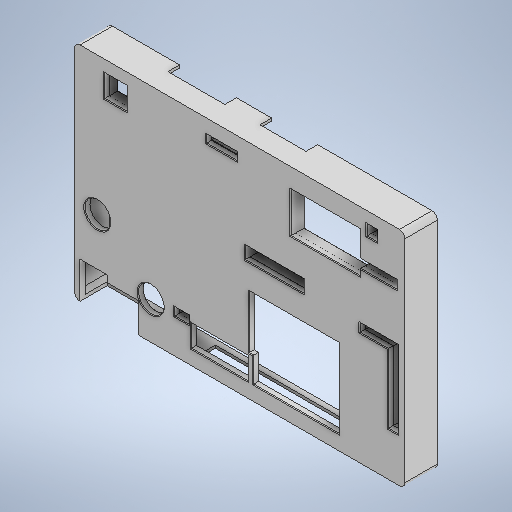
# Autodesk Inventor part: tampa_KiiRA
Saved by Autodesk Inventor 2026.3 (Build 303398000, 398)
## iProperties
Created: 2026-05-20
Part Number: tampa_KiiRA
Material: Genérico
Document SubType Name: Modeling
Designer: franciscowilke
Density: 1 g/cm^3
Appearance: Padrão
Author: franciscowilke
Autodesk Inventor part; units mm, degrees
ref_plane "YZ Plane" through (0, 0, 0) normal (1, 0, 0) x (0, 1, 0)
ref_plane "XZ Plane" through (0, 0, 0) normal (0, 1, 0) x (-1, 0, 0)
ref_plane "XY Plane" through (0, 0, 0) normal (0, 0, 1) x (1, 0, 0)
sketch "Esboço2" plane through (0, 0, 0) normal (0, 0, 1) x (1, 0, 0)
  line L0 (60.2596, 45.3747) -> (-61.7404, 45.3747)
  line L1 (-61.7404, 45.3747) -> (-61.7404, -36.6253)
  line L2 (-61.7404, -36.6253) -> (60.2596, -36.6253)
  line L3 (60.2596, -36.6253) -> (60.2596, 45.3747)
  line L4 (60.2596, 45.3747) -> (-61.7404, -36.6253) construction
  line L5 (-61.7404, 45.3747) -> (60.2596, -36.6253) construction
  point P0 (0, 0)
  dimension "d9" = 122
  dimension "d10" = 82
  constraints: 12 end point, 2 parallel, 1 horizontal, 1 perpendicular
  measures "d9" distance of L2.end L1.end
  measures "d10" distance of L1.end L0.end
extrude "Extrusão6" add sketch "Esboço2" against normal blind 12
sketch "Esboço11" plane through (0, 0, -12) normal (0, 0, -1) x (-1, 0, 0)
  line L0 (61.7404, -36.6253) -> (61.7404, 45.3747) construction
  line L1 (61.7404, 45.3747) -> (-60.2596, 45.3747) construction
  line L2 (-60.2596, 45.3747) -> (-60.2596, -36.6253) construction
  line L3 (-60.2596, -36.6253) -> (61.7404, -36.6253) construction
  line L4 (-60.2596, 45.3747) -> (61.7404, 45.3747)
  line L5 (61.7404, 45.3747) -> (61.7404, -36.6253)
  line L6 (61.7404, -36.6253) -> (-60.2596, -36.6253)
  line L7 (-60.2596, -36.6253) -> (-60.2596, 45.3747)
  line L8 (-59.2596, 44.3747) -> (60.7404, 44.3747)
  line L9 (60.7404, 44.3747) -> (60.7404, -35.6253)
  line L10 (60.7404, -35.6253) -> (-59.2596, -35.6253)
  line L11 (-59.2596, -35.6253) -> (-59.2596, 44.3747)
  point P0 (0, 0)
  dimension "d193" = 1
  constraints: 16 end point, 2 parallel, 1 horizontal, 1 perpendicular, 3 other
  measures "d193" distance between parallel lines of L1 L8
extrude "Extrusão8" cut sketch "Esboço11" against normal blind 10 contours L8 L9 L10 L11
fillet "Arredondamento3" radius 2 8 edges at (-60.7404, 44.3747, -7) (60.2596, -36.6253, -6) (-61.7404, -36.6253, -6) (-60.7404, -35.6253, -7) (-61.7404, 45.3747, -6) (60.2596, 45.3747, -6) (59.2596, 44.3747, -7) (59.2596, -35.6253, -7)
sketch "Esboço4" plane through (0, 0, 0) normal (0, 0, 1) x (1, 0, 0)
  line L0 (2.6091, -2.1634) -> (35.9721, -2.118)
  line L1 (53.9733, -20.4796) -> (53.9372, 5.0204)
  line L2 (53.9372, 5.0204) -> (43.5268, 5.0002)
  line L3 (22.8706, 7.0991) -> (1.1206, 7.0659)
  line L4 (1.1206, 7.0659) -> (1.1206, 11.8159)
  line L5 (1.1206, 11.8159) -> (22.8706, 11.8159)
  line L6 (22.8706, 11.8159) -> (22.8706, 7.0991)
  line L7 (17.9879, 23.1518) -> (43.7379, 23.1518)
  line L8 (43.7379, 23.1518) -> (43.7379, 25.5518)
  circle A0 centre (-53.3326, -5.722) radius 4.75
  arc A1 (-28.9083, -23.3517) -> (-38.3779, -23.3517) centre (-33.6431, -22.972) ccw
  line L9 (17.9879, 23.1518) -> (17.9879, 38.1518)
  line L10 (43.5178, 8.1502) -> (57.7177, 8.191)
  line L11 (-61.7404, -36.6253) -> (-61.7404, 45.3747) construction
  line L12 (-42.5184, 32.6531) -> (-50.7684, 32.6531)
  line L13 (-50.7684, 32.6531) -> (-50.7684, 40.9031)
  line L14 (-50.7684, 40.9031) -> (-42.5184, 40.9031)
  line L15 (-42.5184, 40.9031) -> (-42.5184, 32.6531)
  line L16 (17.9879, 38.1518) -> (43.7379, 38.1518)
  line L17 (57.7177, 8.191) -> (57.7582, -20.4743)
  line L18 (57.7582, -20.4743) -> (53.9733, -20.4796)
  line L19 (43.5268, 5.0002) -> (43.5178, 8.1502)
  line L20 (43.7379, 28.7386) -> (57.2379, 28.7386)
  line L21 (57.2379, 28.7386) -> (57.2379, 25.5518)
  line L22 (57.2379, 25.5518) -> (43.7379, 25.5518)
  line L23 (43.7379, 28.7386) -> (43.7379, 38.1518)
  line L24 (46.0539, 37.0934) -> (50.0539, 37.0934)
  line L25 (50.0539, 37.0934) -> (50.0539, 41.0934)
  line L26 (50.0539, 41.0934) -> (46.0539, 41.0934)
  line L27 (46.0539, 41.0934) -> (46.0539, 37.0934)
  line L28 (-19.4139, -21.0043) -> (-24.9029, -21.0043)
  line L29 (-24.9029, -21.0043) -> (-24.9029, -24.0043)
  line L30 (-24.9029, -24.0043) -> (-19.4139, -24.0043)
  line L31 (-19.4139, -24.0043) -> (-19.4139, -21.0043)
  line L32 (-18.7647, -23.0681) -> (2.1683, -23.0681)
  line L33 (-18.7647, -31.2181) -> (-18.7647, -23.0681)
  circle A2 centre (-33.6431, -22.972) radius 4.75
  line L34 (-1.7534, 40.1185) -> (-13.1034, 40.1185)
  line L35 (-13.1034, 40.1185) -> (-13.1034, 37.2185)
  line L36 (-13.1034, 37.2185) -> (-1.7534, 37.2185)
  line L37 (-1.7534, 37.2185) -> (-1.7534, 40.1185)
  line L38 (35.9721, -31.218) -> (35.9633, -31.218)
  line L39 (35.9764, -22.7351) -> (35.9678, -22.7352)
  line L40 (58.2596, -36.6253) -> (-59.7404, -36.6253) construction
  line L41 (-59.7404, -36.6253) -> (-49.4904, -36.6253)
  line L42 (-49.4904, -36.6253) -> (-49.4904, -23.1253)
  line L43 (-49.4904, -23.1253) -> (-59.7404, -23.1253)
  line L44 (-59.7404, -23.1253) -> (-59.7404, -36.6253)
  line L45 (35.9721, -2.118) -> (35.9721, -31.218)
  line L46 (2.6087, -21.9378) -> (4.2037, -21.9378)
  line L47 (4.2037, -21.9378) -> (4.2035, -31.2181)
  line L48 (2.1683, -23.0681) -> (2.1683, -31.2181)
  line L49 (35.9633, -31.218) -> (4.2035, -31.2181)
  line L50 (2.1683, -31.2181) -> (-18.7647, -31.2181)
  line L51 (2.6091, -2.1634) -> (2.6087, -21.9378)
  point P0 (0, 0)
  point P1 (-38.3779, -23.3517)
  dimension "d132" = 25.5
  dimension "d139" = 3.15
  dimension "d172" = 9.5
  dimension "d173" = 9.5
  dimension "d215" = 25.75
  dimension "d245" = 4.75
  dimension "d246" = 21.75
  dimension "d247" = 14.2
  dimension "d249" = 8.25
  dimension "d250" = 15
  dimension "d251" = 25.75
  dimension "d255" = 9.4133
  dimension "d256" = 8.25
  dimension "d297" = 4
  dimension "d314" = 4
  dimension "d326" = 5.489
  dimension "d327" = 3
  dimension "d342" = 54.728
  dimension "d346" = 11.35
  dimension "d347" = 2.9
  dimension "d349" = 13.5
  dimension "d350" = 10.25
  dimension "d351" = 8.15
  dimension "d353" = 29.1
  dimension "d356" = 1.595
  constraints: 100 end point, 12 perpendicular, 9 parallel, 6 horizontal, 3 centre point, 2 point on circle, 1 coincident, 1 vertical
  measures "d132" distance of L1.start L1.end
  measures "d139" distance of L2.end L10.start
  measures "d172" diameter of A0
  measures "d173" diameter of A1
  measures "d215" distance of L7.start L7.end
  measures "d245" distance of L3.end L4.end
  measures "d246" distance of L3.start L3.end
  measures "d247" distance of L10.start L10.end
  measures "d249" distance of L14.end L12.start
  measures "d250" distance of L7.start L9.end
  measures "d251" distance of L9.end L16.end
  measures "d255" distance of L16.end L20.start
  measures "d256" distance of L13.end L14.end
  measures "d297" distance of L26.end L25.end
  measures "d314" distance of L26.end L24.start
  measures "d326" distance of L29.end L30.end
  measures "d327" distance of L30.end L28.start
  measures "d342" distance of L38.end L33.start
  measures "d346" distance of L34.start L34.end
  measures "d347" distance of L36.end L34.start
  measures "d349" distance of L41.end L42.end
  measures "d350" distance of L42.end L43.end
  measures "d351" distance of L33.start L32.start
  measures "d353" distance of L0.end L38.start
  measures "d356" distance of L46.start L46.end
extrude "Extrusão10" cut sketch "Esboço4" against normal blind 10
sketch "Esboço12" plane through (-59.7404, -36.6253, -12) normal (0, -1, 0) x (1, 0, 0)
  line L0 (118, 0) -> (0, 0) construction
  line L1 (0, 12) -> (21.75, 12)
  line L2 (21.75, 12) -> (21.75, 2)
  line L3 (0, 2) -> (0, 12)
  line L4 (10.25, 12) -> (10.25, 2) construction
  line L5 (21.75, 2) -> (0, 2)
  point P0 (113.7333, 0)
  point P1 (59.7404, 12)
  point P2 (21.75, 0)
  point P3 (10.25, 0)
  point P4 (1.1624, 0)
  dimension "d382" = 2
  constraints: 8 end point, 2 perpendicular, 2 point on line, 1 horizontal, 1 parallel
  measures "d382" distance between parallel lines of L0 L5
extrude "Extrusão11" cut sketch "Esboço12" against normal blind 11
sketch "Esboço13" plane through (-59.7404, 45.3747, 0) normal (0, 1, 0) x (1, 0, 0)
  line L0 (0, 12) -> (118, 12) construction
  line L1 (45.7717, 12) -> (24.7717, 12)
  line L2 (24.7717, 12) -> (24.7717, 7.7)
  line L3 (24.7717, 7.7) -> (45.7717, 7.7)
  line L4 (45.7717, 7.7) -> (45.7717, 12)
  line L5 (1, 12) -> (117, 12) construction
  line L6 (58.7717, 12) -> (75.7717, 12)
  line L7 (75.7717, 12) -> (75.7717, 7.7)
  line L8 (75.7717, 7.7) -> (58.7717, 7.7)
  line L9 (58.7717, 7.7) -> (58.7717, 12)
  point P0 (59.7404, 0)
  point P1 (71.7717, 12)
  point P2 (21.75, 12)
  point P3 (113.7333, 10)
  dimension "d233" = 21
  dimension "d235" = 4.3
  dimension "d241" = 17
  dimension "d243" = 4.3
  dimension "d244" = 13
  constraints: 16 end point, 4 parallel, 2 horizontal, 2 perpendicular, 4 other
  measures "d233" distance of L3.end L2.end
  measures "d235" distance of L3.end L1.start
  measures "d241" distance of L7.end L8.end
  measures "d243" distance of L8.end L6.start
  measures "d244" distance of L1.start L6.start
extrude "Extrusão12" cut sketch "Esboço13" against normal blind 18
sketch "Esboço15" plane through (-61.7404, -34.6253, 0) normal (-1, 0, 0) x (0, 0, 1)
  line L0 (0, 80) -> (-12, 80) construction
  line L1 (-6.2849, 34) -> (-6.2849, 44)
  line L2 (-6.2849, 44) -> (-14.2849, 44)
  line L3 (-14.2849, 44) -> (-14.2849, 34)
  line L4 (-14.2849, 34) -> (-6.2849, 34)
  line L5 (-12, 78) -> (-12, 80) construction
  line L6 (-6.2849, 34) -> (-6.2849, 80)
  point P0 (0, 34.6253)
  dimension "d268" = 8
  dimension "d270" = 46
  dimension "d289" = 10
  constraints: 10 end point, 2 parallel, 2 perpendicular, 1 point on line
  measures "d268" distance of L3.end L1.start
  measures "d270" distance of L1.start L6.end
  measures "d289" distance of L2.end L3.end
extrude "Extrusão14" cut sketch "Esboço15" against normal blind 20
sketch "Esboço16" plane through (58.2596, -36.6253, -12) normal (0, -1, 0) x (1, 0, 0)
  line L0 (0, 0) -> (-118, 0) construction
  line L1 (2, 0) -> (0, 0) construction
  line L2 (2, 0) -> (-4, 0)
  line L3 (-78, 2) -> (-78, 6)
  line L4 (-4, 6) -> (-4, 2)
  line L5 (-18.4636, 6) -> (-18.4636, 2)
  line L6 (-23.4916, 6) -> (-23.4916, 2)
  line L7 (-78, 6) -> (-23.4916, 6)
  line L8 (-23.4916, 2) -> (-78, 2)
  line L9 (-13.1799, 6) -> (-13.1799, 2)
  line L10 (-9.6587, 6) -> (-9.6587, 2)
  line L11 (-18.4636, 6) -> (-13.1799, 6)
  line L12 (-9.6587, 6) -> (-4, 6)
  line L13 (-13.1799, 2) -> (-18.4636, 2)
  line L14 (0, 12) -> (0, 0) construction
  line L15 (-9.6587, 2) -> (-4, 2)
  point P0 (-96.25, 0)
  point P1 (-58.2596, 12)
  dimension "d371" = 4
  dimension "d372" = 54.5084
  dimension "d376" = 5.2838
  dimension "d378" = 4
  dimension "d381" = 6
  constraints: 26 end point, 9 perpendicular, 1 parallel, 1 point on line
  measures "d371" distance of L6.start L6.end
  measures "d372" distance of L3.end L6.start
  measures "d376" distance of L5.start L9.start
  measures "d378" distance of L9.start L9.end
  measures "d381" distance of L4.start L2.end
extrude "Extrusão15" cut sketch "Esboço16" against normal blind 3.871
sketch "Esboço19" plane through (0, 0, -2) normal (0, 0, -1) x (-1, 0, 0)
  line L0 (-57.2379, 25.5518) -> (-57.2379, 28.7386) construction
  line L1 (-57.2379, 28.7386) -> (-43.7379, 28.7386) construction
  line L2 (-43.7379, 28.7386) -> (-43.7379, 38.1518) construction
  line L3 (-43.7379, 38.1518) -> (-17.9879, 38.1518) construction
  line L4 (-17.9879, 38.1518) -> (-17.9879, 23.1518) construction
  line L5 (-17.9879, 23.1518) -> (-43.7379, 23.1518) construction
  line L6 (-43.7379, 23.1518) -> (-43.7379, 25.5518) construction
  line L7 (-43.7379, 25.5518) -> (-57.2379, 25.5518) construction
  line L8 (-50.0539, 41.0934) -> (-46.0539, 41.0934) construction
  line L9 (-46.0539, 41.0934) -> (-46.0539, 37.0934) construction
  line L10 (-46.0539, 37.0934) -> (-50.0539, 37.0934) construction
  line L11 (-50.0539, 37.0934) -> (-50.0539, 41.0934) construction
  line L12 (50.7684, 40.9031) -> (50.7684, 32.6531) construction
  line L13 (50.7684, 32.6531) -> (42.5184, 32.6531) construction
  line L14 (42.5184, 32.6531) -> (42.5184, 40.9031) construction
  line L15 (42.5184, 40.9031) -> (50.7684, 40.9031) construction
  line L16 (-50.0539, 41.0934) -> (-46.0539, 41.0934)
  line L17 (-46.0539, 41.0934) -> (-46.0539, 37.0934)
  line L18 (-46.0539, 37.0934) -> (-50.0539, 37.0934)
  line L19 (-50.0539, 37.0934) -> (-50.0539, 41.0934)
  line L20 (-43.7379, 38.1518) -> (-17.9879, 38.1518)
  line L21 (-17.9879, 38.1518) -> (-17.9879, 23.1518)
  line L22 (-17.9879, 23.1518) -> (-43.7379, 23.1518)
  line L23 (-57.2379, 28.7386) -> (-43.7379, 28.7386)
  line L24 (-43.7379, 25.5518) -> (-57.2379, 25.5518)
  line L25 (-57.2379, 25.5518) -> (-57.2379, 28.7386)
  line L26 (-57.7177, 8.191) -> (-43.5268, 8.191)
  line L27 (-43.5268, 8.191) -> (-43.5268, 5.0002)
  line L28 (-43.5268, 5.0002) -> (-53.9733, 5.0002)
  line L29 (-57.7177, 5.0277) -> (-57.7177, 8.191)
  line L30 (-53.9733, 5.0002) -> (-53.9733, -20.4796)
  line L31 (-53.9733, -20.4796) -> (-57.7177, -20.4796)
  line L32 (-57.7177, -20.4796) -> (-57.7177, 5.0277)
  line L33 (-22.8706, 11.8159) -> (-1.1206, 11.8159)
  line L34 (-1.1206, 11.8159) -> (-1.1206, 7.0659)
  line L35 (-1.1206, 7.0659) -> (-22.8706, 7.0659)
  line L36 (-22.8706, 7.0659) -> (-22.8706, 11.8159)
  line L37 (42.5184, 40.9031) -> (42.5184, 32.6531) construction
  line L38 (42.5184, 40.9031) -> (50.7684, 40.9031)
  line L39 (50.7684, 40.9031) -> (50.7684, 32.6531)
  line L40 (50.7684, 32.6531) -> (42.5184, 32.6531)
  line L41 (42.5184, 32.6531) -> (42.5184, 40.9031)
  line L42 (-43.7379, 23.1518) -> (-43.7379, 25.5518)
  line L43 (-43.7379, 28.7386) -> (-43.7379, 38.1518)
  line L44 (-42.7768, 8.941) -> (-58.4677, 8.941)
  line L45 (-58.4677, 8.941) -> (-58.4677, 5.0277)
  line L46 (-58.4677, 5.0277) -> (-58.4677, -21.2296)
  line L47 (-58.4677, -21.2296) -> (-53.2233, -21.2296)
  line L48 (-53.2233, -21.2296) -> (-53.2233, 4.2502)
  line L49 (-53.2233, 4.2502) -> (-42.7768, 4.2502)
  line L50 (-42.7768, 4.2502) -> (-42.7768, 8.941)
  line L51 (-57.4879, 28.9886) -> (-57.4879, 25.3018)
  line L52 (-57.4879, 25.3018) -> (-43.9879, 25.3018)
  line L53 (-43.9879, 25.3018) -> (-43.9879, 22.9018)
  line L54 (-43.9879, 22.9018) -> (-17.7379, 22.9018)
  line L55 (-17.7379, 22.9018) -> (-17.7379, 38.4018)
  line L56 (-17.7379, 38.4018) -> (-43.9879, 38.4018)
  line L57 (-43.9879, 38.4018) -> (-43.9879, 28.9886)
  line L58 (-43.9879, 28.9886) -> (-57.4879, 28.9886)
  line L59 (-50.3039, 36.8434) -> (-45.8039, 36.8434)
  line L60 (-45.8039, 36.8434) -> (-45.8039, 41.3434)
  line L61 (-45.8039, 41.3434) -> (-50.3039, 41.3434)
  line L62 (-50.3039, 41.3434) -> (-50.3039, 36.8434)
  line L63 (42.2684, 41.1531) -> (42.2684, 32.4031)
  line L64 (42.2684, 32.4031) -> (51.0184, 32.4031)
  line L65 (51.0184, 32.4031) -> (51.0184, 41.1531)
  line L66 (51.0184, 41.1531) -> (42.2684, 41.1531)
  line L67 (-0.8706, 12.0659) -> (-23.1206, 12.0659)
  line L68 (-23.1206, 12.0659) -> (-23.1206, 6.8159)
  line L69 (-23.1206, 6.8159) -> (-0.8706, 6.8159)
  line L70 (-0.8706, 6.8159) -> (-0.8706, 12.0659)
  line L71 (24.9029, -21.0043) -> (19.4139, -21.0043) construction
  line L72 (19.4139, -24.0043) -> (24.9029, -24.0043) construction
  line L73 (19.4139, -21.0043) -> (24.9029, -21.0043)
  line L74 (24.9029, -21.0043) -> (24.9029, -24.0043)
  line L75 (24.9029, -24.0043) -> (19.4139, -24.0043)
  line L76 (19.4139, -24.0043) -> (19.4139, -21.0043)
  line L77 (25.1529, -24.2543) -> (25.1529, -20.7543)
  line L78 (25.1529, -20.7543) -> (19.1639, -20.7543)
  line L79 (19.1639, -20.7543) -> (19.1639, -24.2543)
  line L80 (19.1639, -24.2543) -> (25.1529, -24.2543)
  line L81 (1.7534, 40.1185) -> (1.7534, 37.2185) construction
  line L82 (1.7534, 40.1185) -> (13.0191, 40.1185)
  line L83 (13.0191, 40.1185) -> (13.0191, 37.4185)
  line L84 (13.0191, 37.4185) -> (1.7534, 37.4185)
  line L85 (1.7534, 37.4185) -> (1.7534, 40.1185)
  line L86 (13.2691, 37.1685) -> (13.2691, 40.3685)
  line L87 (13.2691, 40.3685) -> (1.5034, 40.3685)
  line L88 (1.5034, 40.3685) -> (1.5034, 37.1685)
  line L89 (1.5034, 37.1685) -> (13.2691, 37.1685)
  point P0 (0, 0)
  dimension "d317" = 0.75
  dimension "d318" = 0.25
  dimension "d319" = 0.25
  dimension "d320" = 0.25
  dimension "d321" = 0.25
  dimension "d345" = 0.25
  dimension "d348" = 0.25
  constraints: 140 end point, 26 parallel, 11 perpendicular, 8 horizontal, 28 other
  measures "d317" distance between parallel lines of L26 L44
  measures "d318" distance between parallel lines of L0 L51
  measures "d319" distance between parallel lines of L10 L59
  measures "d320" distance between parallel lines of L14 L63
  measures "d321" distance between parallel lines of L33 L67
  measures "d345" distance between parallel lines of L74 L77
  measures "d348" distance between parallel lines of L83 L86
extrude "Extrusão18" add sketch "Esboço19" along normal blind 3
chamfer "Chanfro3" distance 0.25 angle 45 46 edges at (-46.6434, 40.9031, 0) (-42.5184, 36.7781, 0) (-46.6434, 32.6531, 0) (-50.7684, 36.7781, 0) (-7.4284, 37.2185, 0) (-13.1034, 38.6685, 0) (-7.4284, 40.1185, 0) (-1.7534, 38.6685, 0) (48.0539, 37.0934, 0) (50.0539, 39.0934, 0) (48.0539, 41.0934, 0) (46.0539, 39.0934, 0) (30.8629, 38.1518, 0) (43.7379, 33.4452, 0) (50.4879, 28.7386, 0) (57.2379, 27.1452, 0) (50.4879, 25.5518, 0) (43.7379, 24.3518, 0) (30.8629, 23.1518, 0) (17.9879, 30.6518, 0) (11.9956, 7.0825, 0) (1.1206, 9.4409, 0) (11.9956, 11.8159, 0) (22.8706, 9.4575, 0) (50.6177, 8.1706, 0) (48.732, 5.0103, 0) (53.9552, -7.7296, 0) (57.738, -6.1417, 0) (55.8657, -20.4769, 0) (-58.0826, -5.722, 0) (-28.9083, -22.5923, 0) (-22.1584, -24.0043, 0) (-19.4139, -22.5043, 0) (-22.1584, -21.0043, 0) (-24.9029, -22.5043, 0) (-18.7647, -27.1431, 0) (-8.2982, -23.0681, 0) (-8.2982, -31.2181, 0) (2.1683, -27.1431, 0) (4.2036, -26.5779, 0) (20.0834, -31.218, 0) (3.4062, -21.9378, 0) (2.6089, -12.0506, 0) (19.2906, -2.1407, 0) (35.9721, -16.668, 0) (43.5223, 6.5752, 0)
